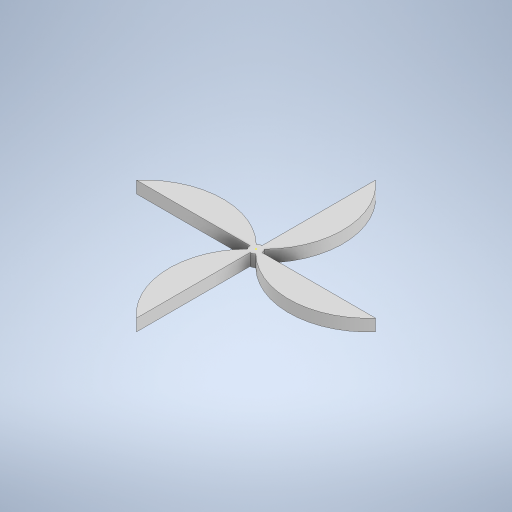
# Autodesk Inventor part: fan_num4_1
Saved by Autodesk Inventor 2024 (Build 280153000, 153)
## iProperties
Created: 2024-08-06
Part Number: fan_num4_1
Material: 일반
Document SubType Name: Modeling
Designer: chlqj
Density: 1 g/cm^3
Appearance: 기본값
Author: chlqj
Autodesk Inventor part; units mm, degrees
ref_plane "YZ Plane" through (0, 0, 0) normal (1, 0, 0) x (0, 1, 0)
ref_plane "XZ Plane" through (0, 0, 0) normal (0, 1, 0) x (-1, 0, 0)
ref_plane "XY Plane" through (0, 0, 0) normal (0, 0, 1) x (1, 0, 0)
sketch "스케치6" plane through (0, 0, 0) normal (0, 1, 0) x (-1, 0, 0)
  circle A0 centre (0, 0) radius 15
  dimension "d16" = 30
  constraints: 1 centre point, 1 coincident
  measures "d16" diameter of A0
extrude "돌출4" add sketch "스케치6" along normal blind 1.5
sketch "스케치7" plane through (0, 1.5, 0) normal (0, 1, 0) x (1, 0, 0)
  circle A0 centre (0, 0) radius 15 projected
  arc A1 (0, 0) -> (-15, 0) centre (-7.5, -6.6144) ccw
  arc A2 (0, 0) -> (0, 15) centre (-6.6144, 7.5) ccw
  arc A3 (0, 0) -> (15, 0) centre (7.5, 6.6144) ccw
  arc A4 (0, 0) -> (0, -15) centre (6.6144, -7.5) ccw
  line L0 (0, -15) -> (0, 0)
  line L1 (0, 0) -> (15, 0)
  line L2 (0, 0) -> (0, 15)
  line L3 (0, 0) -> (-15, 0)
  arc A5 (-15, 0) -> (0, -15) centre (0, 0) ccw
  arc A6 (0, -15) -> (15, 0) centre (0, 0) ccw
  arc A7 (15, 0) -> (0, 15) centre (0, 0) ccw
  arc A8 (0, 15) -> (-15, 0) centre (0, 0) ccw
  point P0 (0, -15)
  point P1 (0, -15)
  dimension "d19" = 10
  dimension "d20" = 10
  dimension "d21" = 10
  dimension "d22" = 10
  dimension "d23" = 15
  dimension "d24" = 15
  constraints: 19 point on circle, 8 centre point, 8 end point, 4 concentric, 3 perpendicular, 1 vertical
  measures "d19" radius of A1
  measures "d20" radius of A2
  measures "d21" radius of A3
  measures "d22" radius of A4
  measures "d23" distance of L0.end L3.end
  measures "d24" distance of L0.start L0.end
extrude "돌출5" cut sketch "스케치7" against normal blind 1.5 contours L1 A2 A0 | A0 L0 A3 | L2 A1 A0 | A0 L3 A4
sketch "스케치8" plane through (0, 1.5, 0) normal (0, 1, 0) x (1, 0, 0)
  arc A0 (0, 0) -> (0, -15) centre (6.6144, -7.5) ccw projected
  circle A1 centre (0, 0) radius 0.75
  dimension "d27" = 1.5
  constraints: 1 centre point, 1 coincident
  measures "d27" diameter of A1
extrude "돌출6" add sketch "스케치8" against normal blind 1.5
sketch "스케치9" plane through (0, 1.5, 0) normal (0, 1, 0) x (1, 0, 0)
  point P0 (0, 0)
